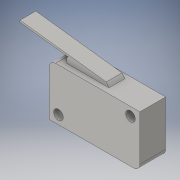
# Autodesk Inventor part: switch
Saved by Autodesk Inventor 2016 (Build 200138000, 138)
## iProperties
Created: 2016-02-16
Part Number: switch
Material: Generic
Document SubType Name: Modeling
Designer: jforce
Density: 1 g/cm^3
Appearance: Default
Author: jforce
Autodesk Inventor part; units mm, degrees
ref_plane "YZ Plane" through (0, 0, 0) normal (1, 0, 0) x (0, 1, 0)
ref_plane "XZ Plane" through (0, 0, 0) normal (0, 1, 0) x (-1, 0, 0)
ref_plane "XY Plane" through (0, 0, 0) normal (0, 0, 1) x (1, 0, 0)
sketch "Sketch1" plane through (0, 0, 0) normal (0, 0, 1) x (1, 0, 0)
  line L0 (0, 61.5875) -> (62, 61.5875) construction
  line L1 (62, 61.5875) -> (62, -0.4125) construction
  line L2 (62, -0.4125) -> (0, -0.4125) construction
  line L3 (0, -0.4125) -> (0, 61.5875) construction
  line L4 (20.3147, 23.8321) -> (46.4322, 23.8321)
  line L5 (48.4322, 25.8321) -> (48.4322, 39.9079)
  line L6 (20.3147, 37.9079) -> (20.3147, 23.8321)
  line L7 (24.0433, 41.0082) -> (24.0433, 39.9079)
  line L8 (26.2438, 41.0082) -> (26.2438, 39.9079)
  line L9 (24.0433, 39.9079) -> (22.3147, 39.9079)
  line L10 (8.8232, 7.7562) -> (58.8232, 7.7562)
  line L11 (9.5567, 44.2478) -> (36.2683, 41.0082)
  line L12 (9.4874, 43.6764) -> (9.5567, 44.2478)
  line L13 (36.1934, 40.391) -> (36.4777, 39.9079)
  line L14 (36.2683, 41.0082) -> (37.1955, 39.9079)
  line L15 (48.4322, 39.9079) -> (37.1955, 39.9079)
  line L16 (36.4777, 39.9079) -> (26.2438, 39.9079)
  arc A0 (26.2438, 41.0082) -> (26.0216, 41.6711) centre (25.1436, 41.0082) ccw
  arc A1 (24.4494, 41.8618) -> (24.0433, 41.0082) centre (25.1436, 41.0082) ccw
  line L17 (36.199, 40.4368) -> (26.0216, 41.6711)
  line L18 (24.4494, 41.8618) -> (9.4874, 43.6764)
  arc A2 (22.3147, 39.9079) -> (20.3147, 37.9079) centre (22.3147, 37.9079) ccw
  arc A3 (46.4322, 23.8321) -> (48.4322, 25.8321) centre (46.4322, 25.8321) ccw
  circle A4 centre (23.179, 26.4983) radius 1.5
  circle A5 centre (45.5157, 37.2749) radius 1.5
  point P0 (0, 0)
  dimension "d9" = 62
  dimension "d16" = 50
  dimension "d18" = 2
  dimension "d19" = 3
  dimension "d20" = 3
  dimension "d27" = 28.1175
  constraints: 30 end point, 8 point on circle, 7 perpendicular, 6 centre point, 6 parallel, 6 tangent, 2 horizontal, 1 equal radius, 2 other
  measures "d9" distance between parallel lines of L1 L3
  measures "d16" distance of L10.start L10.end
  measures "d18" radius of A2
  measures "d19" diameter of A4
  measures "d20" diameter of A5
  measures "d27" distance between parallel lines of L5 L6
extrude "Extrusion2" add sketch "Sketch1" along normal blind 8
sketch "Sketch2" plane through (48.4322, 25.8321, 0) normal (1, 0, 0) x (0, 0, -1)
  line L0 (0, 14.0759) -> (-8, 14.0759) projected
  line L1 (-6.3015, 14.0759) -> (-6.3015, 19.195)
  line L2 (-6.3015, 19.195) -> (-1.4016, 19.195)
  line L3 (-1.4016, 19.195) -> (-1.4016, 14.0759)
  line L4 (-1.4016, 14.0759) -> (1.865, 14.0759)
  line L5 (1.865, 14.0759) -> (1.865, 21.4964)
  line L6 (1.865, 21.4964) -> (-9.1226, 21.4964)
  line L7 (-9.1226, 21.4964) -> (-9.1226, 14.0759)
  line L8 (-9.1226, 14.0759) -> (-6.3015, 14.0759)
  point P0 (0, -25.8321)
  constraints: 16 end point, 6 perpendicular, 3 point on line, 1 horizontal, 1 vertical
extrude "Extrusion3" cut sketch "Sketch2" against normal through all contours L0 L3 L2 L1 L8 L7 L6 L5 L4
body "Solid2"
